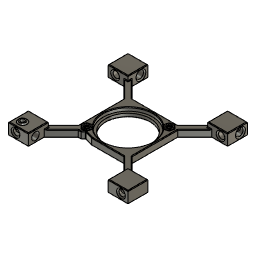
bottom_stepper_holder v10 (Autodesk Fusion 360 design; units mm, degrees)
Autodesk Fusion 360 part; units mm, degrees
note: some values were not read from the file. Chosen so that the rebuilt part matches the saved one: which face or edge a step refers to; which pieces of a blend or face edit are solid. Set by a fixed rule: which sketch regions a step uses.
sketch "Sketch1" plane through (0, 0, 0) normal (0, 0, 1) x (1, 0, 0)
  line L0 (-17.5716, -17.5716) -> (17.5716, 17.5716) construction
  line L1 (17.5716, 17.5716) -> (-17.5716, 17.5716) construction
  line L2 (-17.5716, 17.5716) -> (17.5716, -17.5716) construction
  line L3 (17.5716, -17.5716) -> (-17.5716, -17.5716) construction
  line L4 (-17.5716, 17.5716) -> (-17.5716, -17.5716) construction
  line L5 (17.5716, 17.5716) -> (17.5716, -17.5716) construction
  line L6 (21.15, -21.15) -> (21.15, 21.15)
  line L7 (21.15, 21.15) -> (-21.15, 21.15)
  circle A0 centre (0, 0) radius 21.15
  line L8 (-21.15, 21.15) -> (-21.15, -21.15)
  line L9 (-21.15, -21.15) -> (21.15, -21.15)
  line L10 (23, 23) -> (-23, 23)
  line L11 (-23, 23) -> (-23, -23)
  line L12 (-23, -23) -> (23, -23)
  line L13 (23, -23) -> (23, 23)
  line L14 (23, 23) -> (-23, -23) construction
  line L15 (-23, 23) -> (23, -23) construction
  circle A1 centre (17.5714, 17.5716) radius 1.75
  circle A2 centre (-17.5716, -17.5714) radius 1.75
  dimension "d20" = 42.3
  dimension "d21" = 46
  dimension "d22" = 46
  constraint horizontal L1
  constraint parallel L1 L3
  constraint perpendicular L3 L4
  constraint perpendicular L3 L5
  constraint vertical L6
  constraint horizontal L7
  constraint midpoint L2 A0.centre
  constraint perpendicular L3 L8
  constraint perpendicular L6 L9
  constraint horizontal L10
  constraint perpendicular L10 L11
  constraint parallel L10 L12
  constraint parallel L11 L13
  constraint coincident L14 A0.centre
  constraint coincident L15 A0.centre
  constraint coincident A0.centre origin
  measures "d20" diameter of A0
  measures "d21" distance of L11.end L12.end
  measures "d22" distance of L10.end L11.end
extrude "Extrude1" add sketch "Sketch1" along normal blind 6 contours L6 A0 L9 | L6 L7 A0 | A0 L8 L9 | L7 A0 L8 | L10 L11 L12 L13
extrude "Extrude2" add sketch "Sketch1" along normal blind 3 contours A0
sketch "Sketch2" plane through (0, 0, 0) normal (0, 0, -1) x (1, 0, 0)
  line L0 (23, -23) -> (23, 23)
  line L1 (23, 23) -> (-23, 23)
  line L2 (-23, 23) -> (-23, -23)
  line L3 (-23, -23) -> (23, -23)
  line L4 (-14.6716, 19.2459) -> (-17.5716, 20.9202)
  line L5 (-17.5716, 20.9202) -> (-20.4716, 19.2459)
  line L6 (-20.4716, 19.2459) -> (-20.4716, 15.8973)
  line L7 (-20.4716, 15.8973) -> (-17.5716, 14.223)
  line L8 (-17.5716, 14.223) -> (-14.6716, 15.8973)
  line L9 (-14.6716, 15.8973) -> (-14.6716, 19.2459)
  line L10 (17.5714, 20.9202) -> (14.6714, 19.2459)
  line L11 (20.4714, 19.2459) -> (17.5714, 20.9202)
  line L12 (20.4714, 15.8973) -> (20.4714, 19.2459)
  line L13 (17.5714, 14.223) -> (20.4714, 15.8973)
  line L14 (14.6714, 15.8973) -> (17.5714, 14.223)
  line L15 (14.6714, 19.2459) -> (14.6714, 15.8973)
  line L16 (-17.5716, -14.2228) -> (-20.4716, -15.8971)
  line L17 (-14.6716, -15.8971) -> (-17.5716, -14.2228)
  line L18 (-14.6716, -19.2457) -> (-14.6716, -15.8971)
  line L19 (-17.5716, -20.92) -> (-14.6716, -19.2457)
  line L20 (-20.4716, -19.2457) -> (-17.5716, -20.92)
  line L21 (-20.4716, -15.8971) -> (-20.4716, -19.2457)
  line L22 (17.5714, -14.2228) -> (14.6714, -15.8971)
  line L23 (20.4714, -15.8971) -> (17.5714, -14.2228)
  line L24 (20.4714, -19.2457) -> (20.4714, -15.8971)
  line L25 (17.5714, -20.92) -> (20.4714, -19.2457)
  line L26 (14.6714, -19.2457) -> (17.5714, -20.92)
  line L27 (14.6714, -15.8971) -> (14.6714, -19.2457)
  circle A0 centre (17.5714, -17.5716) radius 1.75
  circle A1 centre (-17.5716, 17.5714) radius 1.75
  point P0 (-17.5716, 17.5716)
  dimension "d27" = 2.9
  dimension "d30" = 35.143
  dimension "d31" = -35.143
  measures "d27" distance of P0 L9
extrude "Extrude3" cut sketch "Sketch2" against normal blind 5 contours L4 L5 L6 L7 L8 L9 | L22 L23 L24 L25 L26 L27 | A0 | A1
sketch "Sketch3" plane through (0, 0, 3) normal (0, 0, 1) x (-1, 0, 0)
  circle A0 centre (0, 0) radius 21.15
  circle A1 centre (0, 0) radius 19
  dimension "d38" = 38
  constraint coincident A0.centre A1.centre
  measures "d38" diameter of A1
extrude "Extrude4" cut sketch "Sketch3" against normal blind 5 contours A1
extrude "Extrude5" add sketch "Sketch1" along normal blind 0.2 from surface at 5 contours A1 | A2
sketch "Sketch5" plane through (0, 0, 6) normal (0, 0, 1) x (-1, 0, 0)
  circle A0 centre (17.5716, 17.5714) radius 1.75
  circle A1 centre (-17.5714, -17.5716) radius 1.75
  circle A2 centre (0, 0) radius 21.15
  line L0 (-23, -23) -> (23, -23)
  line L1 (23, -23) -> (23, 23)
  line L2 (23, 23) -> (-23, 23)
  line L3 (-23, 23) -> (-23, -23)
  line L4 (23, 13.2097) -> (8, 13.2097) construction
  line L5 (8, 13.2097) -> (8, 23) construction
  line L6 (23, 13.2097) -> (15, 13.2097) construction
  line L7 (15, 23) -> (15, 13.2097) construction
  line L8 (15, 23) -> (15, 21) construction
  line L9 (15, 23) -> (15, 21)
  line L10 (8, 23) -> (15, 21)
  line L11 (15, 23) -> (8, 23)
  dimension "d57" = 15
  dimension "d58" = 8
  dimension "d59" = 2
  constraint coincident L1 L4.start
  constraint perpendicular L3 L4
  constraint coincident L2 L5.end
  constraint perpendicular L2 L5
  constraint coincident L4 L6.end
  constraint coincident L2 L7.start
  constraint perpendicular L6 L7
  constraint coincident L7 L8.end
  measures "d57" distance of L4.start L4.end
  measures "d58" distance of L4.start L6.end
  measures "d59" distance of L7.start L8.end
extrude "Extrude7" cut sketch "Sketch5" against normal blind 21 contours L2 L9 L10 L11
chamfer "Chamfer1" distance 2 distance2 2 1 edges at (-15, -23, 3) measured on face at (-20.3333, -23, 2)
fillet "Fillet6" radius 0.5 2 edges at (-15, -21.0004, 3) (-15, -21, 3)
sketch "Sketch6" plane through (0, 0, 0) normal (0, 0, 1) x (1, 0, 0)
  line L0 (0, 23) -> (0, 51) construction
  line L1 (-23, 23) -> (-23, -23) construction
  line L2 (50, 50) -> (-50, 50) construction
  line L3 (-50, 50) -> (-50, -50) construction
  line L4 (-50, -50) -> (50, -50) construction
  line L5 (50, -50) -> (50, 50) construction
  line L6 (50, 50) -> (-50, -50) construction
  line L7 (-50, 50) -> (50, -50) construction
  line L8 (-50, 50) -> (-40, 50)
  line L9 (-40, 50) -> (-40, 40)
  line L10 (-40, 40) -> (-50, 40)
  line L11 (-50, 40) -> (-50, 50)
  line L12 (-50, 40) -> (-40, 50) construction
  line L13 (-23, 23) -> (23, -23) construction
  line L14 (71.5494, 71.5494) -> (-71.5494, -71.5494) construction
  line L15 (-46.7678, 43.2322) -> (-1.7678, -1.7678)
  arc A0 (-1.7678, -1.7678) -> (1.7678, 1.7678) centre (0, 0) ccw
  line L16 (1.7678, 1.7678) -> (-43.2322, 46.7678)
  arc A1 (-43.2322, 46.7678) -> (-46.7678, 43.2322) centre (-45, 45) ccw
  line L17 (-45, 45) -> (0, 0) construction
  line L18 (-40, -40) -> (-40, -50)
  line L19 (-40, -50) -> (-50, -50)
  line L20 (-50, -50) -> (-50, -40)
  line L21 (-50, -40) -> (-40, -40)
  arc A2 (-46.7678, -43.2322) -> (-43.2322, -46.7678) centre (-45, -45) ccw
  line L22 (-40, -50) -> (-50, -40) construction
  line L23 (-43.2322, -46.7678) -> (1.7678, -1.7678)
  line L24 (-1.7678, 1.7678) -> (-46.7678, -43.2322)
  arc A3 (1.7678, -1.7678) -> (-1.7678, 1.7678) centre (0, 0) ccw
  line L25 (40, -40) -> (50, -40)
  line L26 (50, -40) -> (50, -50)
  line L27 (50, -50) -> (40, -50)
  line L28 (40, -50) -> (40, -40)
  arc A4 (43.2322, -46.7678) -> (46.7678, -43.2322) centre (45, -45) ccw
  line L29 (50, -40) -> (40, -50) construction
  line L30 (46.7678, -43.2322) -> (1.7678, 1.7678)
  line L31 (-1.7678, -1.7678) -> (43.2322, -46.7678)
  arc A5 (1.7678, 1.7678) -> (-1.7678, -1.7678) centre (0, 0) ccw
  line L32 (40, 40) -> (40, 50)
  line L33 (40, 50) -> (50, 50)
  line L34 (50, 50) -> (50, 40)
  line L35 (50, 40) -> (40, 40)
  arc A6 (46.7678, 43.2322) -> (43.2322, 46.7678) centre (45, 45) ccw
  line L36 (40, 50) -> (50, 40) construction
  line L37 (43.2322, 46.7678) -> (-1.7678, 1.7678)
  line L38 (1.7678, -1.7678) -> (46.7678, 43.2322)
  arc A7 (-1.7678, 1.7678) -> (1.7678, -1.7678) centre (0, 0) ccw
  line L39 (23, 23) -> (-23, 23)
  line L40 (-23, 23) -> (-23, -23)
  line L41 (-23, -23) -> (23, -23)
  line L42 (23, -23) -> (23, 23)
  line L43 (23, 23) -> (-23, -23) construction
  line L44 (-23, 23) -> (23, -23) construction
  line L45 (-39, 51) -> (-51, 51)
  line L46 (-51, 51) -> (-51, 39)
  line L47 (-51, 39) -> (-39, 39)
  line L48 (-39, 39) -> (-39, 51)
  line L49 (-39, 51) -> (-51, 39) construction
  line L50 (-51, 51) -> (-39, 39) construction
  line L51 (-39, -39) -> (-51, -39)
  line L52 (-51, -39) -> (-51, -51)
  line L53 (-51, -51) -> (-39, -51)
  line L54 (-39, -51) -> (-39, -39)
  line L55 (39, -39) -> (39, -51)
  line L56 (39, -51) -> (51, -51)
  line L57 (51, -51) -> (51, -39)
  line L58 (51, -39) -> (39, -39)
  line L59 (39, 39) -> (51, 39)
  line L60 (51, 39) -> (51, 51)
  line L61 (51, 51) -> (39, 51)
  line L62 (39, 51) -> (39, 39)
  line L63 (-51, -51) -> (-34, -51)
  line L64 (-34, -51) -> (-34, -34)
  line L65 (-34, -34) -> (-51, -34)
  line L66 (-51, -34) -> (-51, -51)
  line L67 (51, -51) -> (34, -51)
  line L68 (34, -51) -> (34, -34)
  line L69 (34, -34) -> (51, -34)
  line L70 (51, -34) -> (51, -51)
  line L71 (-51, 51) -> (-34, 51)
  line L72 (-34, 51) -> (-34, 34)
  line L73 (-34, 34) -> (-51, 34)
  line L74 (-51, 34) -> (-51, 51)
  line L75 (51, 51) -> (34, 51)
  line L76 (34, 51) -> (34, 34)
  line L77 (34, 34) -> (51, 34)
  line L78 (51, 34) -> (51, 51)
  point P0 (-45, 45)
  dimension "d69" = 28
  dimension "d98" = 100
  dimension "d99" = 100
  dimension "d100" = 10
  dimension "d101" = 10
  dimension "d105" = 5
  dimension "d107" = 360
  dimension "d108" = 46
  dimension "d109" = 46
  dimension "d154" = 12
  dimension "d155" = 12
  dimension "d157" = 360
  dimension "d190" = 17
  dimension "d191" = 17
  dimension "d192" = 17
  dimension "d193" = 17
  dimension "d194" = 17
  dimension "d195" = 17
  dimension "d196" = 17
  dimension "d197" = 17
  constraint horizontal L2
  constraint perpendicular L2 L3
  constraint parallel L2 L4
  constraint parallel L3 L5
  constraint coincident L6 A0.centre
  constraint coincident L7 A0.centre
  constraint coincident A0.centre L17.end
  constraint horizontal L8
  constraint vertical L9
  constraint horizontal L10
  constraint vertical L11
  constraint coincident L13 A0.centre
  constraint coincident L14 A0.centre
  constraint tangent L15 A0
  constraint tangent A0 L16
  constraint parallel L15 L16
  constraint tangent L16 A1
  constraint tangent L15 A1
  constraint perpendicular L14 L17
  constraint midpoint L12 P0
  constraint horizontal L39
  constraint perpendicular L39 L40
  constraint parallel L39 L41
  constraint parallel L40 L42
  constraint coincident L43 A0.centre
  constraint coincident L44 A0.centre
  constraint horizontal L45
  constraint perpendicular L45 L46
  constraint parallel L45 L47
  constraint parallel L46 L48
  constraint coincident L49 P0
  constraint coincident L50 P0
  constraint coincident P0 A1.centre
  constraint horizontal L63
  constraint vertical L64
  constraint horizontal L65
  constraint vertical L66
  constraint horizontal L67
  constraint vertical L68
  constraint horizontal L69
  constraint vertical L70
  constraint horizontal L71
  constraint vertical L72
  constraint horizontal L73
  constraint vertical L74
  constraint horizontal L75
  constraint vertical L76
  constraint horizontal L77
  constraint vertical L78
  measures "d69" distance of L0.start L0.end
  measures "d98" distance of L3.end L4.end
  measures "d99" distance of L2.end L3.end
  measures "d100" distance of L2.end L8.end
  measures "d101" distance of L2.end L10.end
  measures "d105" diameter of A0
  measures "d108" distance of L1.end L13.end
  measures "d109" distance of L1.start L1.end
  measures "d154" distance of L46.end L47.end
  measures "d155" distance of L45.end L46.end
  measures "d190" distance of L52.end L63.end
  measures "d191" distance of L52.end L65.end
  measures "d192" distance of L56.end L67.end
  measures "d193" distance of L56.end L69.end
  measures "d194" distance of L45.end L71.end
  measures "d195" distance of L45.end L73.end
  measures "d196" distance of L60.end L75.end
  measures "d197" distance of L60.end L77.end
extrude "Extrude11" add sketch "Sketch6" along normal blind 6 contours L9 L10 L15 L16 L47 L48 | L15 L16 L47 L48 L72 L73 | L15 L16 L39 L40 L72 L73 | L37 L38 L39 L42 L76 L77 | L23 L24 L40 L41 L64 L65 | L37 L38 L59 L62 L76 L77 | L23 L24 L51 L54 L64 L65 | L32 L35 L37 L38 L59 L62 | L18 L21 L23 L24 L51 L54 | L30 L31 L41 L42 L68 L69 | L30 L31 L55 L58 L68 L69 | L25 L28 L30 L31 L55 L58
extrude "Extrude12" add sketch "Sketch6" along normal blind 10 contours L8 L9 L10 L11 L15 L16 L45 L46 L47 L48 L71 L74 | L8 L9 L10 L11 L15 L16 A1 | L9 L10 L15 L16 L47 L48 | L9 L10 L15 L16 A1 | L16 L48 L71 L72 | L15 L16 L47 L48 L72 L73 | L15 L47 L73 L74 | L37 L62 L75 L76 | L37 L38 L59 L62 L76 L77 | L23 L24 L51 L54 L64 L65 | L24 L51 L65 L66 | L32 L33 L34 L35 L37 L38 L59 L60 L61 L62 L75 L78 | L32 L35 L37 L38 L59 L62 | L18 L21 L23 L24 L51 L54 | L18 L19 L20 L21 L23 L24 L51 L52 L53 L54 L63 L66 | L32 L35 A6 L37 L38 | L32 L33 L34 L35 A6 L37 L38 | L38 L59 L77 L78 | L18 L19 L20 L21 A2 L23 L24 | L18 L21 A2 L23 L24 | L23 L54 L63 L64 | L30 L58 L69 L70 | L30 L31 L55 L58 L68 L69 | L31 L55 L67 L68 | L25 L26 L27 L28 L30 L31 L55 L56 L57 L58 L67 L70 | L25 L28 L30 L31 L55 L58 | L25 L28 A4 L30 L31 | L25 L26 L27 L28 A4 L30 L31
sketch "Sketch9" plane through (51, 0, 0) normal (1, 0, 0) x (0, 1, 0)
  line L0 (-50, 0) -> (-40, 0)
  line L1 (-40, 0) -> (-40, 10)
  line L2 (-40, 10) -> (-50, 10)
  line L3 (-50, 10) -> (-50, 0)
  line L4 (-50, 0) -> (-40, 10) construction
  line L5 (-50, 10) -> (-40, 0) construction
  line L6 (-50, 10) -> (50, 10) construction
  line L7 (50, 10) -> (50, 0) construction
  line L8 (50, 0) -> (40, 0) construction
  line L9 (40, 0) -> (50, 10) construction
  line L10 (50, 0) -> (40, 10) construction
  circle A0 centre (-45, 5) radius 3.25
  circle A1 centre (45, 5) radius 3.25
  line L11 (-51, 0) -> (-34, 0)
  line L12 (-34, 10) -> (-51, 10)
  line L13 (-51, 10) -> (-51, 0)
  line L14 (-34, 0) -> (-34, 10)
  dimension "d128" = 100
  dimension "d129" = 10
  dimension "d130" = 10
  dimension "d131" = 6.5
  dimension "d132" = 6.5
  constraint coincident L0.start L3.end
  constraint coincident L1.end L2.start
  constraint coincident L2.end L3.start
  constraint coincident L0.end L1.start
  constraint perpendicular L3 L6
  constraint perpendicular L6 L7
  constraint perpendicular L3 L8
  constraint coincident L6 L10.end
  constraint perpendicular L9 L10
  constraint midpoint L5 A0.centre
  constraint midpoint L10 A1.centre
  measures "d128" distance of L2.end L6.end
  measures "d129" distance of L6.end L7.end
  measures "d130" distance of L7.end L8.end
  measures "d131" diameter of A0
  measures "d132" diameter of A1
sketch "Sketch10" plane through (0, 51, 0) normal (0, 1, 0) x (-1, 0, 0)
  line L0 (-50, 0) -> (-40, 0)
  line L1 (-40, 0) -> (-40, 10)
  line L2 (-40, 10) -> (-50, 10)
  line L3 (-50, 10) -> (-50, 0)
  line L4 (-50, 0) -> (-40, 10) construction
  line L5 (-50, 10) -> (-40, 0) construction
  line L6 (-50, 10) -> (50, 10) construction
  line L7 (50, 10) -> (50, 0) construction
  line L8 (50, 0) -> (40, 0) construction
  line L9 (40, 0) -> (50, 10) construction
  line L10 (50, 0) -> (40, 10) construction
  circle A0 centre (45, 5) radius 2.75
  circle A1 centre (-45, 5) radius 2.75
  line L11 (-51, 0) -> (-34, 0)
  line L12 (-34, 10) -> (-51, 10)
  line L13 (-51, 10) -> (-51, 0)
  line L14 (-34, 0) -> (-34, 10)
  dimension "d133" = 100
  dimension "d134" = 10
  dimension "d135" = 10
  dimension "d136" = 5.5
  dimension "d137" = 5.5
  constraint coincident L0.start L3.end
  constraint coincident L1.end L2.start
  constraint coincident L2.end L3.start
  constraint coincident L0.end L1.start
  constraint perpendicular L3 L6
  constraint perpendicular L6 L7
  constraint perpendicular L7 L8
  constraint coincident L6 L10.end
  constraint perpendicular L9 L10
  constraint midpoint L10 A0.centre
  constraint midpoint L5 A1.centre
  measures "d133" distance of L2.end L6.end
  measures "d134" distance of L6.end L7.end
  measures "d135" distance of L7.end L8.end
  measures "d136" diameter of A0
  measures "d137" diameter of A1
extrude "Extrude14" cut sketch "Sketch9" against normal blind 102 contours A0 | A1
extrude "Extrude15" cut sketch "Sketch10" against normal blind 102 contours A0 | A1
sketch "Sketch11" plane through (0, 0, 6) normal (0, 0, 1) x (-1, 0, 0)
  line L0 (-34, -37.5355) -> (-19.4645, -23)
  line L1 (-19.4645, -23) -> (19.4645, -23)
  line L2 (19.4645, -23) -> (34, -37.5355)
  line L3 (37.5355, -34) -> (23, -19.4645)
  line L4 (23, -19.4645) -> (23, 19.4645)
  line L5 (23, 19.4645) -> (37.5355, 34)
  line L6 (34, 37.5355) -> (19.4645, 23)
  line L7 (19.4645, 23) -> (17, 23)
  line L8 (17, 23) -> (15.208, 21.208)
  arc A0 (14.7171, 21.0808) -> (15.208, 21.208) centre (14.8545, 21.5616) ccw
  line L9 (14.7171, 21.0808) -> (8, 23)
  line L10 (8, 23) -> (-19.4645, 23)
  line L11 (-19.4645, 23) -> (-34, 37.5355)
  line L12 (-37.5355, 34) -> (-23, 19.4645)
  line L13 (-23, 19.4645) -> (-23, -19.4645)
  line L14 (-23, -19.4645) -> (-37.5355, -34)
  circle A1 centre (0, 0) radius 21.15
  circle A2 centre (17.5716, 17.5714) radius 1.75
  circle A3 centre (-17.5714, -17.5716) radius 1.75
  line L15 (20.3744, 14.7176) -> (21.4445, 18.5718)
  line L16 (21.4445, 18.5718) -> (18.6417, 21.4256)
  line L17 (18.6417, 21.4256) -> (14.7688, 20.4252)
  line L18 (14.7688, 20.4252) -> (13.6987, 16.571)
  line L19 (13.6987, 16.571) -> (16.5015, 13.7172)
  line L20 (16.5015, 13.7172) -> (20.3744, 14.7176)
  line L21 (-20.4745, -14.8198) -> (-21.406, -18.7098)
  line L22 (-21.406, -18.7098) -> (-18.503, -21.4616)
  line L23 (-18.503, -21.4616) -> (-14.6683, -20.3234)
  line L24 (-14.6683, -20.3234) -> (-13.7368, -16.4334)
  line L25 (-13.7368, -16.4334) -> (-16.6398, -13.6816)
  line L26 (-16.6398, -13.6816) -> (-20.4745, -14.8198)
  line L27 (-34, 34) -> (-37.5355, 34)
  line L28 (-37.5355, -34) -> (-34, -34)
  line L29 (-34, -34) -> (-34, -37.5355)
  line L30 (34, -37.5355) -> (34, -34)
  line L31 (34, -34) -> (37.5355, -34)
  line L32 (37.5355, 34) -> (34, 34)
  line L33 (34, 34) -> (34, 37.5355)
  line L34 (-34, 37.5355) -> (-34, 34)
  point P0 (17.5716, 17.5714)
  point P1 (-17.5714, -17.5716)
  dimension "d148" = 4
  dimension "d149" = 4
  constraint coincident P0 A2.centre
  constraint coincident P1 A3.centre
  measures "d148" distance of L15.start P0
  measures "d149" distance of L21.start P1
chamfer "Chamfer20" distance 0.5 angle 45 1 faces at (-25.4882, 25.4882, 6)
extrude "Extrude16" add sketch "Sketch11" along normal blind 1 contours L15 L16 L17 L18 L19 L20 | L21 L22 L23 L24 L25 L26
ref_plane "WorkPlane1" through (17, 0, 3.25) normal (1, 0, 0) x (0, 1, 0)
chamfer "Chamfer13" distance 0.5 angle 45 2 faces at (-18.279, -14.7667, 7) (16.7844, 20.3542, 7)
extrude "Extrude28" add sketch "Sketch10" against normal blind 2 contours A0 | A1
extrude "Extrude29" add sketch "Sketch9" against normal blind 2 contours A0
extrude "Extrude30" add sketch "Sketch9" along normal blind 2 from surface at -102 contours A1
chamfer "Chamfer17" distance 1 angle 45 8 edges at (-51, -48.0301, 3.8247) (-42.4361, -51, 4.0056) (-42.4361, 34, 4.0056) (34, -48.0301, 3.8247) (47.5639, -51, 4.0056) (47.5639, 34, 4.0056) (51, 41.9699, 6.1753) (-34, 41.9699, 6.1753)
sketch "Sketch13" plane through (0, 0, 10) normal (0, 0, 1) x (-1, 0, 0)
  line L0 (51, 34) -> (51, 51)
  line L1 (51, 51) -> (34, 51)
  line L2 (34, 51) -> (34, 34)
  line L3 (34, 34) -> (51, 34)
  line L4 (51, 51) -> (39, 39) construction
  line L5 (51, 51) -> (39, 51) construction
  circle A0 centre (45, 45) radius 1.75
  circle A1 centre (45, 45) radius 2.75
  dimension "d206" = 45
  dimension "d207" = 16.9706
  dimension "d208" = 3.5
  dimension "d211" = 5.5
  constraint horizontal L5
  constraint coincident L0.end L1.start
  constraint midpoint L4 A0.centre
  constraint concentric A0 A1
  measures "d206" angle of L4 L5
  measures "d207" distance of L0.end L4.end
  measures "d208" diameter of A0
  measures "d211" diameter of A1
extrude "Extrude31" cut sketch "Sketch13" against normal blind 9 contours A0
extrude "Extrude32" add sketch "Sketch13" along normal blind 1 contours A1
extrude "Extrude33" cut 2 faces at (-14.998, -15.3652, 6) (15.4027, 14.9609, 6) along direction (0, 0, 1) blind 3.5
chamfer "Chamfer18" distance 1 angle 45 1 edges at (-42.4361, -45.9944, 10)
chamfer "Chamfer19" distance 0.5 angle 45 1 faces at (-46.5118, -39.6667, 0)
chamfer "Chamfer21" distance 0.5 angle 45 4 edges at (-42.5, -51, 10) (-34, -42.5, 10) (-42.5, -34, 10) (-51, -42.5, 10) 3 faces at (-45.3333, 45.3333, 10) (45.3333, 45.3333, 10) (45.3333, -45.3333, 10)
equation "d27 = ( 5.8 / 2 ) * 1 mm"
equation "d98 = outer_cube_width"
equation "d99 = outer_cube_width"
equation "outer_cube_width = 100 mm"
equation "d128 = outer_cube_width"
equation "d133 = outer_cube_width"
equation "d207 = ( ( 2 * 12 ^ 2 ) ^ 0.5 ) * 1 mm"
named bodies: "bottom_stepper_holder"
